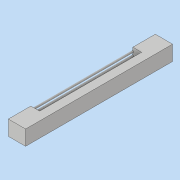
# Autodesk Inventor part: support
Saved by Autodesk Inventor 2019 (Build 230136000, 136)
## iProperties
Created: 2020-02-20
Part Number: support
Material: Generic
Document SubType Name: Modeling
Designer: Sudhanshu
Density: 1 g/cm^3
Appearance: Default
Author: Sudhanshu
Autodesk Inventor part; units mm, degrees
ref_plane "YZ Plane" through (0, 0, 0) normal (1, 0, 0) x (0, 1, 0)
ref_plane "XZ Plane" through (0, 0, 0) normal (0, 1, 0) x (-1, 0, 0)
ref_plane "XY Plane" through (0, 0, 0) normal (0, 0, 1) x (1, 0, 0)
sketch "Sketch1" plane through (0, 0, 0) normal (1, 0, 0) x (0, 1, 0)
  line L0 (0, 0) -> (-100, 0)
  line L1 (-100, 0) -> (-100, -150)
  line L2 (-100, -150) -> (0, -150)
  line L3 (0, -150) -> (0, 0)
  dimension "d0" = 100
  dimension "d1" = 150
  constraints: 8 end point, 2 parallel, 1 horizontal, 1 perpendicular
  measures "d0" distance of L2.end L1.end
  measures "d1" distance of L1.end L0.end
extrude "Extrusion1" add sketch "Sketch1" along normal blind 15
sketch "Sketch2" plane through (0, -100, 0) normal (0, 0, 1) x (1, 0, 0)
  line L0 (0, 100) -> (0, 0) projected
  line L1 (0, 100) -> (0, 0)
  line L2 (0, 0) -> (0, 19)
  line L3 (0, 100) -> (0, 81)
  line L4 (0, 81) -> (0, 75)
  line L5 (0, 75) -> (0, 69)
  circle A0 centre (0, 75) radius 6
  line L6 (0, 69) -> (0, 56)
  line L7 (0, 56) -> (0, 50)
  circle A1 centre (0, 50) radius 6
  line L8 (0, 44) -> (0, 31)
  line L9 (0, 31) -> (0, 25)
  circle A2 centre (0, 25) radius 6
  dimension "d11" = 12
  dimension "d4" = 19
  dimension "d5" = 19
  dimension "d6" = 6
  dimension "d7" = 6
  dimension "d8" = 12
  dimension "d9" = 13
  dimension "d10" = 6
  dimension "d12" = 13
  dimension "d13" = 6
  dimension "d14" = 12
  constraints: 16 end point, 3 coincident, 2 centre point, 1 vertical alignment, 14 other
  measures "d4" distance of L0.end L2.end
  measures "d5" distance of L0.start L3.end
  measures "d6" distance of L3.end L4.end
  measures "d7" distance of L4.end L5.end
  measures "d8" diameter of A0
  measures "d9" distance of L5.end L6.end
  measures "d10" distance of L6.end L7.end
  measures "d12" distance of L8.start L8.end
  measures "d13" distance of L8.end L9.end
  measures "d14" diameter of A2
extrude "Extrusion2" add sketch "Sketch2" along normal blind 680
sketch "Sketch3" plane through (0, -25, 680) normal (0, 0, 1) x (1, 0, 0)
  line L0 (0, -75) -> (0, 25) projected
  line L1 (15, 25) -> (15, -75) projected
  line L2 (0, 25) -> (15, 25)
  line L3 (15, 25) -> (15, -75)
  line L4 (15, -75) -> (0, -75)
  line L5 (0, -75) -> (0, 25)
  constraints: 8 end point, 2 parallel, 1 horizontal, 1 perpendicular
extrude "Extrusion3" add sketch "Sketch3" along normal blind 150
sketch "Sketch4" plane through (15, -100, 680) normal (1, 0, 0) x (0, 0, -1)
  line L0 (0, 100) -> (-150, 100) projected
  line L1 (830, 0) -> (830, 100) projected
  line L2 (-150, 100) -> (830, 100)
  line L3 (830, 100) -> (830, 0)
  line L4 (830, 0) -> (-150, 0)
  line L5 (-150, 0) -> (-150, 100)
  point P0 (680, 100)
  constraints: 8 end point, 2 parallel, 1 horizontal, 1 perpendicular
extrude "Extrusion4" add sketch "Sketch4" along normal blind 100
sketch "Sketch5" plane through (0, 0, 0) normal (0, 1, 0) x (1, 0, 0)
  line L0 (15, -680) -> (0, -680) projected
  line L1 (15, -680) -> (58.7284, -680)
  line L2 (58.7284, -680) -> (58.7284, 0)
  line L3 (58.7284, 0) -> (15, 0)
  line L4 (15, 0) -> (15, -680)
  point P0 (0, 0)
  constraints: 8 end point, 2 parallel, 1 horizontal, 1 perpendicular
extrude "Extrusion5" cut sketch "Sketch5" along normal through all both and the other way through all
body "Solid1"
